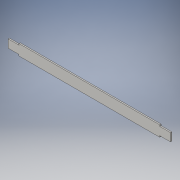
# Autodesk Inventor part: back
Saved by Autodesk Inventor 2016 SP2 (Build 200236200, 236)
## iProperties
Created: 2017-09-04
Part Number: back
Material: Generic
Document SubType Name: Modeling
Designer: Kartikye
Density: 1 g/cm^3
Appearance: Default
Author: Kartikye
Autodesk Inventor part; units mm, degrees
ref_plane "YZ Plane" through (0, 0, 0) normal (1, 0, 0) x (0, 1, 0)
ref_plane "XZ Plane" through (0, 0, 0) normal (0, 1, 0) x (-1, 0, 0)
ref_plane "XY Plane" through (0, 0, 0) normal (0, 0, 1) x (1, 0, 0)
sketch "Sketch1" plane through (0, 0, 0) normal (0, 0, 1) x (1, 0, 0)
  line L0 (0, 7.9375) -> (-165.1, 7.9375)
  line L1 (-165.1, 7.9375) -> (-165.1, 4.7625)
  line L2 (-165.1, 4.7625) -> (-190.5, 4.7625)
  line L3 (-190.5, 4.7625) -> (-190.5, -14.0589)
  line L4 (-190.5, -14.0589) -> (-165.1, -14.0589)
  line L5 (-165.1, -14.0589) -> (-165.1, -17.2339)
  line L6 (-165.1, -17.2339) -> (165.1, -17.2339)
  line L7 (165.1, -17.2339) -> (165.1, -14.0589)
  line L8 (165.1, -14.0589) -> (190.5, -14.0589)
  line L9 (190.5, -14.0589) -> (190.5, 4.7625)
  line L10 (190.5, 4.7625) -> (165.1, 4.7625)
  line L11 (165.1, 4.7625) -> (165.1, 7.9375)
  line L12 (165.1, 7.9375) -> (0, 7.9375)
  point P0 (0, 0)
  dimension "d0" = 165.1
  dimension "d1" = 3.175
  dimension "d2" = 25.4
  dimension "d3" = 18.8214
  dimension "d4" = 25.4
  dimension "d5" = 3.175
  dimension "d6" = 330.2
  dimension "d7" = 3.175
  dimension "d8" = 25.4
  dimension "d9" = 90
  dimension "d10" = 18.8214
  dimension "d11" = 25.4
  dimension "d12" = 3.175
  constraints: 26 end point, 6 point on line, 5 perpendicular, 1 horizontal
  measures "d0" distance of L0.start L0.end
  measures "d1" distance of L0.end L1.end
  measures "d2" distance of L1.end L2.end
  measures "d3" distance of L2.end L3.end
  measures "d4" distance of L3.end L4.end
  measures "d5" distance of L4.end L5.end
  measures "d6" distance of L5.end L6.end
  measures "d7" distance of L6.end L7.end
  measures "d8" distance of L7.end L8.end
  measures "d9" angle of L7 L8
  measures "d10" distance of L8.end L9.end
  measures "d11" distance of L9.end L10.end
  measures "d12" distance of L10.end L11.end
extrude "Extrusion1" add sketch "Sketch1" along normal blind 3.175
body "Solid1"
